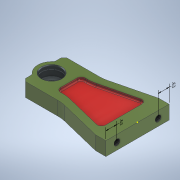
# Autodesk Inventor part: bearing holder
Saved by Autodesk Inventor 2020 (Build 240168000, 168)
## iProperties
Created: 2020-08-07
Part Number: bearing holder
Material: Iron, Ductile
Document SubType Name: Modeling
Designer: benny
Density: 7.15 g/cm^3
Appearance: Iron Gray
Author: benny
Autodesk Inventor part; units mm, degrees
ref_plane "YZ Plane" through (0, 0, 0) normal (1, 0, 0) x (0, 1, 0)
ref_plane "XZ Plane" through (0, 0, 0) normal (0, 1, 0) x (-1, 0, 0)
sketch "Sketch1" plane through (0, 0, 0) normal (0, 1, 0) x (-1, 0, 0)
  line L0 (0, 46) -> (0, -46)
  line L1 (0, -46) -> (15, -46)
  line L2 (15, -46) -> (15, -30)
  line L3 (15, -30) -> (80, -30)
  line L4 (80, -30) -> (15, -46)
  line L5 (15, -30) -> (80, -30)
  line L6 (80, -30) -> (133, -30)
  line L7 (133, -30) -> (133, -26)
  line L8 (133, -26) -> (137, -26)
  line L9 (137, -26) -> (133, -30)
  line L10 (133, -26) -> (137, -26)
  line L11 (137, -26) -> (137, 26)
  line L12 (137, 26) -> (133, 26)
  line L13 (133, 26) -> (133, 30)
  line L14 (133, 30) -> (137, 26)
  line L15 (133, 30) -> (80, 30)
  line L16 (80, 30) -> (15, 30)
  line L17 (15, 30) -> (15, 46)
  line L18 (15, 46) -> (80, 30)
  line L19 (15, 46) -> (0, 46)
  line L20 (0, 0) -> (125, 0)
  circle A0 centre (125, 0) radius 20
  point P0 (137, 16)
  point P1 (137, -16)
  dimension "d0" = 92
  dimension "d1" = 15
  dimension "d2" = 16
  dimension "d3" = 65
  dimension "d4" = 53
  dimension "d5" = 4
  dimension "d6" = 4
  dimension "d7" = 52
  dimension "d8" = 4
  dimension "d9" = 4
  dimension "d10" = 53
  dimension "d11" = 65
  dimension "d12" = 16
  dimension "d13" = 125
  dimension "d14" = 40
  constraints: 42 end point, 7 perpendicular, 5 point on line, 2 collinear, 1 centre point, 1 coincident, 1 parallel, 1 vertical
  measures "d0" distance of L0.start L0.end
  measures "d1" distance of L0.end L1.end
  measures "d2" distance of L1.end L2.end
  measures "d3" distance of L2.end L3.end
  measures "d4" distance of L3.end L6.end
  measures "d5" distance of L6.end L7.end
  measures "d6" distance of L7.end L8.end
  measures "d7" distance of L8.end L11.end
  measures "d8" distance of L11.end L12.end
  measures "d9" distance of L12.end L13.end
  measures "d10" distance of L13.end L15.end
  measures "d11" distance of L15.end L16.end
  measures "d12" distance of L16.end L17.end
  measures "d13" distance of L20.start L20.end
  measures "d14" diameter of A0
extrude "Extrusion1" add sketch "Sketch1" along normal blind 20
fillet "Fillet1" radius 5 2 edges at (-137, 10, 16) (-137, 10, -16)
fillet "Fillet2" radius 50 2 edges at (-80, 10, -30) (-80, 10, 30)
sketch "Sketch2" plane through (0, 20, 0) normal (0, 1, 0) x (1, 0, 0)
  line L0 (0, 0) -> (-20, 0)
  line L1 (-20, 0) -> (-20, 34)
  line L2 (-20, 34) -> (-20, 18)
  line L3 (-20, 18) -> (-85, 18)
  line L4 (-85, 18) -> (-20, 34)
  line L5 (-85, 18) -> (-100, 18)
  line L6 (-100, 18) -> (-100, -18)
  line L7 (-100, -18) -> (-85, -18)
  line L8 (-85, -18) -> (-20, -18)
  line L9 (-20, -18) -> (-20, 0)
  line L10 (-20, -18) -> (-20, -34)
  line L11 (-20, -34) -> (-85, -18)
  dimension "d19" = 20
  dimension "d20" = 34
  dimension "d21" = 16
  dimension "d22" = 65
  dimension "d23" = 15
  dimension "d24" = 36
  dimension "d25" = 15
  dimension "d26" = 65
  dimension "d27" = 16
  constraints: 24 end point, 4 perpendicular, 4 point on line, 1 horizontal
  measures "d19" distance of L0.start L0.end
  measures "d20" distance of L0.end L1.end
  measures "d21" distance of L1.end L2.end
  measures "d22" distance of L2.end L3.end
  measures "d23" distance of L3.end L5.end
  measures "d24" distance of L5.end L6.end
  measures "d25" distance of L6.end L7.end
  measures "d26" distance of L7.end L8.end
  measures "d27" distance of L8.end L10.end
extrude "Extrusion2" cut sketch "Sketch2" against normal blind 4
ref_plane "Work Plane1" through (0, 10, 0) normal (0, 1, 0) x (1, 0, 0)
fillet "Fillet3" radius 50 2 edges at (-85, 18, 18) (-85, 18, -18)
fillet "Fillet4" radius 2 8 edges at (-85.0441, 16, 18.3636) (-95.5317, 16, 18) (-49.5562, 16, 26.7246) (-20, 16, 0) (-100, 16, 0) (-49.5562, 16, -26.7246) (-95.5317, 16, -18) (-85.0441, 16, -18.3636)
fillet "Fillet5" radius 6 8 edges at (-100, 19, 18) (-99.4142, 16.5858, 17.4142) (-100, 19, -18) (-99.4142, 16.5858, -17.4142) (-20, 19, 34) (-20.5858, 16.5858, 33.2525) (-20.5858, 16.5858, -33.2525) (-20, 19, -34)
mirror "Mirror1" about plane through (0, 10, 0) normal (0, 1, 0) of "Extrusion2", "Fillet3", "Fillet4", "Fillet5"
sketch "Sketch3" plane through (0, 20, 0) normal (0, 1, 0) x (1, 0, 0)
  line L0 (0, 0) -> (-125, 0)
  circle A0 centre (-125, 0) radius 14
  dimension "d34" = 125
  dimension "d35" = 28
  constraints: 2 end point, 1 centre point, 1 coincident, 1 horizontal
  measures "d34" distance of L0.start L0.end
  measures "d35" diameter of A0
extrude "Extrusion3" cut sketch "Sketch3" against normal blind 14
sketch "Sketch4" plane through (0, 20, 0) normal (0, 1, 0) x (1, 0, 0)
  circle A0 centre (-125, 0) radius 15
  point P0 (0, 0)
  dimension "d38" = 30
  constraints: 1 centre point
  measures "d38" diameter of A0
extrude "Extrusion4" cut sketch "Sketch4" against normal blind 6
sketch "Sketch5" plane through (0, 20, 0) normal (0, 1, 0) x (1, 0, 0)
  circle A0 centre (-125, 0) radius 15
  point P0 (0, 0)
  dimension "d41" = 30
  constraints: 1 centre point
  measures "d41" diameter of A0
extrude "Extrusion5" add sketch "Sketch5" against normal blind 4.5
sketch "Sketch6" plane through (0, 20, 0) normal (0, 1, 0) x (1, 0, 0)
  circle A0 centre (-125, 0) radius 14
  point P0 (0, 0)
  dimension "d44" = 28
  constraints: 1 centre point
  measures "d44" diameter of A0
extrude "Extrusion6" cut sketch "Sketch6" against normal blind 4.5
sketch "Sketch7" plane through (0, 20, 0) normal (0, 1, 0) x (1, 0, 0)
  circle A0 centre (-125, 0) radius 15
  point P0 (0, 0)
  dimension "d47" = 30
  constraints: 1 centre point
  measures "d47" diameter of A0
extrude "Extrusion7" cut sketch "Sketch7" against normal blind 1
chamfer "Chamfer1" distance 1 distance2 1 1 edges at (-140, 19, 0) measured on face at (-110.0486, 19.3333, 1.207)
sketch "Sketch8" plane through (0, 0, 0) normal (0, -1, 0) x (1, 0, 0)
  circle A0 centre (-125, 0) radius 6.5
  point P0 (0, 0)
  dimension "d53" = 13
  constraints: 1 centre point
  measures "d53" diameter of A0
extrude "Extrusion8" cut sketch "Sketch8" against normal blind 6
sketch "Sketch9" plane through (0, 0, 46) normal (1, 0, 0) x (0, 0, -1)
  line L0 (76, 10) -> (111.0219, 10)
  line L1 (92, 0) -> (77.4493, 0) projected
  point P0 (46, 0)
  constraints: 2 end point, 1 parallel
hole "Hole1" at (0, 10, -30) direction (-1, 0, 0) diameter 8.376 depth 20 tip angle 118 thread size "M10x1.5" class "6H" standard "ISO Metric profile"
mirror "Mirror2" about plane through (0, 0, 0) normal (0, 0, 1) of "Hole1"
sketch "Sketch10" plane through (0, 20, 0) normal (0, 1, 0) x (1, 0, 0)
  point P0 (0, 0)
body "Solid1"
